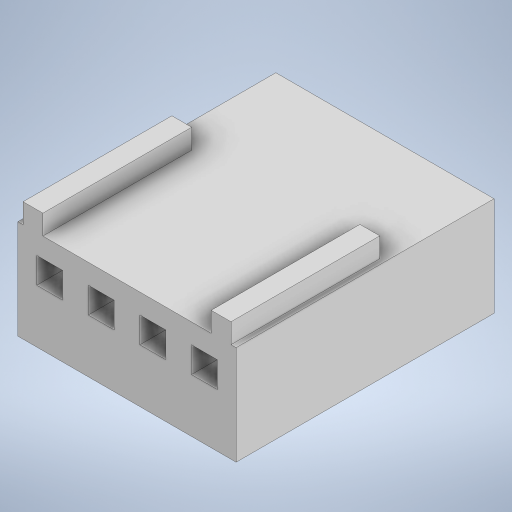
# Autodesk Inventor part: Four-Pin-Shell
Saved by Autodesk Inventor 2023 (Build 270158000, 158)
## iProperties
Created: 2024-03-02
Part Number: Four-Pin-Shell
Material: Generic
Document SubType Name: Modeling
Designer: ongyu
Density: 1 g/cm^3
Appearance: Default
Author: ongyu
Autodesk Inventor part; units mm, degrees
ref_plane "YZ Plane" through (0, 0, 0) normal (1, 0, 0) x (0, 1, 0)
ref_plane "XZ Plane" through (0, 0, 0) normal (0, 1, 0) x (-1, 0, 0)
ref_plane "XY Plane" through (0, 0, 0) normal (0, 0, 1) x (1, 0, 0)
sketch "Sketch1" plane through (0, 0, 0) normal (0, 1, 0) x (-1, 0, 0)
  line L0 (5.5, 6.5) -> (-5.5, 6.5)
  line L1 (-5.5, 6.5) -> (-5.5, -6.5)
  line L2 (-5.5, -6.5) -> (5.5, -6.5)
  line L3 (5.5, -6.5) -> (5.5, 6.5)
  line L4 (0, -9.1) -> (0, 9.1) projected
  line L5 (-7.7, 0) -> (7.7, 0) projected
  point P0 (0, 0)
  dimension "d0" = 11
  dimension "d1" = 5.5
  dimension "d2" = 13
  dimension "d3" = 6.5
  constraints: 8 end point, 2 parallel, 1 horizontal, 1 perpendicular
  measures "d0" distance between parallel lines of L1 L3
  measures "d1" distance between parallel lines of L4 L3
  measures "d2" distance between parallel lines of L2 L0
  measures "d3" distance between parallel lines of L0 L5
extrude "Extrusion1" add sketch "Sketch1" along normal blind 5
sketch "Sketch2" plane through (0, 5, 0) normal (0, 1, 0) x (1, 0, 0)
  line L0 (-5.5, -6.5) -> (5.5, -6.5) projected
  line L1 (-5.24, -6.5) -> (-4.24, -6.5)
  line L2 (-4.24, -6.5) -> (-4.24, 1)
  line L3 (-4.24, 1) -> (-5.24, 1)
  line L4 (-5.24, 1) -> (-5.24, -6.5)
  line L5 (5.24, -6.5) -> (4.24, -6.5)
  line L6 (4.24, -6.5) -> (4.24, 1)
  line L7 (4.24, 1) -> (5.24, 1)
  line L8 (5.24, 1) -> (5.24, -6.5)
  line L9 (5.5, -6.5) -> (5.5, 6.5) projected
  line L10 (-5.5, 6.5) -> (-5.5, -6.5) projected
  point P0 (0, 0)
  point P1 (4.74, 1)
  point P2 (4.24, -6.5)
  dimension "d6" = 0.26
  dimension "d7" = 0.26
  dimension "d8" = 1
  dimension "d9" = 1
  dimension "d10" = 7.5
  dimension "d11" = 7.5
  constraints: 16 end point, 4 parallel, 2 horizontal, 2 perpendicular, 2 point on line, 1 midpoint
  measures "d6" distance between parallel lines of L9 L8
  measures "d7" distance between parallel lines of L10 L4
  measures "d8" distance between parallel lines of L4 L2
  measures "d9" distance between parallel lines of L8 L6
  measures "d10" distance between parallel lines of L0 L3
  measures "d11" distance from line of L0 point (4.74, 1)
extrude "Extrusion2" add sketch "Sketch2" along normal blind 1
sketch "Sketch3" plane through (-5.5, 0, 6.5) normal (0, 0, 1) x (1, 0, 0)
  line L0 (0.95, 4) -> (2.25, 4)
  line L1 (2.25, 4) -> (2.25, 2.7)
  line L2 (2.25, 2.7) -> (0.95, 2.7)
  line L3 (0.95, 2.7) -> (0.95, 4)
  line L4 (3.55, 4) -> (4.85, 4)
  line L5 (4.85, 4) -> (4.85, 2.7)
  line L6 (4.85, 2.7) -> (3.55, 2.7)
  line L7 (3.55, 2.7) -> (3.55, 4)
  line L8 (6.15, 4) -> (7.45, 4)
  line L9 (7.45, 4) -> (7.45, 2.7)
  line L10 (7.45, 2.7) -> (6.15, 2.7)
  line L11 (6.15, 2.7) -> (6.15, 4)
  line L12 (8.75, 4) -> (10.05, 4)
  line L13 (10.05, 4) -> (10.05, 2.7)
  line L14 (10.05, 2.7) -> (8.75, 2.7)
  line L15 (8.75, 2.7) -> (8.75, 4)
  line L16 (0, 0) -> (0, 5) projected
  line L17 (5.5, 7.2) -> (5.5, -1.2) projected
  line L18 (1.26, 5) -> (9.74, 5) projected
  point P0 (5.5, 0)
  point P1 (0.95, 3.35)
  dimension "d14" = 1.3
  dimension "d15" = 1.3
  dimension "d18" = 1.3
  dimension "d19" = 1.3
  dimension "d21" = 1.3
  dimension "d22" = 1.3
  dimension "d23" = 1.3
  dimension "d24" = 0.65
  dimension "d25" = 1.3
  dimension "d26" = 1
  constraints: 32 end point, 8 parallel, 6 point on line, 4 horizontal, 4 perpendicular, 1 midpoint
  measures "d14" distance between parallel lines of L15 L13
  measures "d15" distance between parallel lines of L11 L9
  measures "d18" distance between parallel lines of L3 L1
  measures "d19" distance between parallel lines of L5 L7
  measures "d21" distance between parallel lines of L7 L1
  measures "d22" distance between parallel lines of L15 L9
  measures "d23" distance between parallel lines of L11 L5
  measures "d24" distance between parallel lines of L5 L17
  measures "d25" distance between parallel lines of L14 L12
  measures "d26" distance between parallel lines of L18 L4
extrude "Extrusion3" cut sketch "Sketch3" against normal up to surface (13 mm away)
equation "\"d1\" = 0.5 * d0"
equation "\"d3\" = 0.5 * d2"
equation "\"d7\" = d6"
equation "\"d9\" = d8"
equation "\"d11\" = d10"
equation "\"d15\" = d14"
equation "\"d18\" = d15"
equation "\"d19\" = d18"
equation "\"d21\" = d19"
equation "\"d22\" = d14"
equation "\"d23\" = d15"
equation "\"d24\" = 0.5 * d19"
equation "\"d25\" = d14"
body "Solid1"
